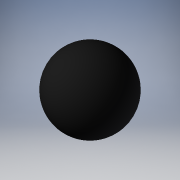
# Autodesk Inventor part: 6007DDU Ball
Saved by Autodesk Inventor 2023 (Build 270158000, 158)
## iProperties
Created: 2023-07-20
Part Number: 6007DDU Ball
Material: Generic
Catalog Web Link: www.cadenas.de
Description: contact_sealed_type_dd_ddu_B-NSK
Vendor: NSK_RB
Document SubType Name: Modeling
Designer: psAdmin
Manufacturer: NSK_RB
Mass: 0.161031 g
Surface Area: 1.43139 cm^2
Volume: 0.161031 cm^3
Density: 1 g/cm^3
Appearance: PSOLRGB-128-128-128
Category: PARTsolutions
Company: NSK_RB
PSOL_IDENT_0: {$CADENAS_DATA/23d-libs/nsk_rb/roller_bearings/deep_groove_bb/single_row_dgbb/contact_sealed_type_dd
PSOL_IDENT_1: _ddu_2_b.prj},188 {VTYP=3D},{NB=6007DDU Ball},{LINA=6007DDU Ball},{NN=contact_sealed_type_dd_ddu_B},
PSOL_IDENT_2: {DATE=15.09.2022 00:32:48},{GEOMDATE=18.05.2018 11:37:08},{VERSION=},{LINEID=1980},{WBVAR=},{WBNUMER
PSOL_IDENT_3: IC=}  {NB=6007DDU Ball},{LINA=6007DDU Ball},{KT=DUMMY},{IDNR=21},{STAN=Standard},{ORDER=6007DDU},{SD=
PSOL_IDENT_4: 35},{X=35},{DI1=43.50},{DI2=41.6},{SDE1=54.10},{SDE2=56.00},{D=62},{DD=62},{B=14},{R=1.0},{CR1=16000
PSOL_IDENT_5: },{COR1=10300},{CR2=1630},{COR2=1050},{FO=14.8},{LG=6700},{A=2.08},{BB=1.90},{DD1=59.61},{RO=0.60},{
PSOL_IDENT_6: RN=0.5},{DD2=67.7},{F=1.70},{DAM1=40.0},{DA1=41.5},{DA2=57.0},{RA=1.0},{DX=68.5},{CY=3.4},{MASS=0.15
PSOL_IDENT_7: 1},{SC=1}
NB: 6007DDU Ball
NN: contact_sealed_type_dd_ddu_B
NT: NSK
NBSYN: $ORDER. Ball
LINA: 6007DDU Ball
CATALOG: NSK Rolling Bearing
IDNR: 21
STAN: Standard
ORDER: 6007DDU
SD: 35
X: 35
DI1: 43.5
DI2: 41.6
SDE1: 54.1
SDE2: 56
D: 62
DD: 62
B: 14
R: 1
CR1: 16000
COR1: 10300
CR2: 1630
COR2: 1050
FO: 14.8
LG: 6700
A: 2.08
BB: 1.9
DD1: 59.61
RO: 0.6
RN: 0.5
DD2: 67.7
F: 1.7
DAM1: 40
DA1: 41.5
DA2: 57
RA: 1
DX: 68.5
CY: 3.4
MASS: 0.151
SC: 1
SUPPLIER: NSK_RB
ARTICLENO: 6007DDU Ball
BOMINFO: 6007DDU Ball
CREATOR: CADENAS GmbH
Title: 6007DDU Ball
Author: Cadenas PARTsolutions
Comments: NSK
Autodesk Inventor part; units mm, degrees
sketch "Sketch_1" plane through (0, 0, 0) normal (0, 0, 1) x (1, 0, 0)
  line L0 (3.375, 0) -> (-3.375, 0)
  arc A0 (3.375, 0) -> (-3.375, 0) centre (0, 0) ccw
  line L1 (3.375, 0) -> (-3.375, 0)
  constraints: 4 end point, 2 point on circle, 1 centre point
revolve "Revolution1" add sketch "Sketch_1" angle 360 about axis through (3.375, 0, 0) along (1, 0, 0)
ref_plane "ip_cst_2_b_1_XY" through (0, 0, 0) normal (1, 0, 0) x (0, 0, -1)
ref_plane "ip_cst_2_b_1_YZ" through (0, 0, 0) normal (0, 0, -1) x (0, 1, 0)
ref_plane "ip_cst_2_b_1_ZX" through (0, 0, 0) normal (0, 1, 0) x (1, 0, 0)
body "Solid1"
